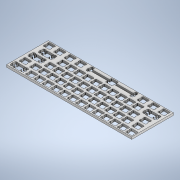
# Autodesk Inventor part: plate
Saved by Autodesk Inventor 2022 (Build 260153000, 153)
## iProperties
Created: 2022-03-01
Part Number: plate
Material: Generic
Document SubType Name: Modeling
Designer: Nathan Griffith
Density: 1 g/cm^3
Appearance: Default
Author: Nathan Griffith
Autodesk Inventor part; units mm, degrees
(part 1 of 2)
ref_plane "YZ Plane" through (0, 0, 0) normal (1, 0, 0) x (0, 1, 0)
ref_plane "XZ Plane" through (0, 0, 0) normal (0, 1, 0) x (-1, 0, 0)
ref_plane "XY Plane" through (0, 0, 0) normal (0, 0, 1) x (1, 0, 0)
sketch "Sketch1" plane through (0, 0, 0) normal (0, 1, 0) x (-1, 0, 0)
  line L0 (0.0951, 95.5075) -> (285.845, 95.5075)
  line L1 (285.845, 95.5075) -> (285.845, 0.2577)
  line L2 (285.845, 0.2577) -> (0.0951, 0.2577)
  line L3 (0.0951, 0.2577) -> (0.0951, 95.5075)
  line L4 (124.062, 16.7831) -> (124.062, 15.7827)
  line L5 (124.062, 15.7827) -> (123.263, 15.7827)
  line L6 (123.263, 15.7827) -> (123.263, 12.6848)
  line L7 (123.263, 12.6848) -> (124.062, 12.6848)
  line L8 (124.062, 12.6848) -> (124.062, 12.0826)
  line L9 (124.062, 12.0826) -> (84.4381, 12.0826)
  line L10 (84.4381, 12.0826) -> (84.4381, 15.3128)
  line L11 (84.4381, 15.3128) -> (82.7126, 15.3128)
  line L12 (82.7126, 15.3128) -> (82.7126, 16.2347)
  line L13 (82.7126, 16.2347) -> (79.412, 16.2347)
  line L14 (79.412, 16.2347) -> (79.412, 15.3128)
  line L15 (79.412, 15.3128) -> (77.687, 15.3128)
  line L16 (77.687, 15.3128) -> (77.687, 12.0826)
  line L17 (77.687, 12.0826) -> (76.8629, 12.0826)
  line L18 (76.8629, 12.0826) -> (76.8629, 9.2838)
  line L19 (76.8629, 9.2838) -> (77.687, 9.2838)
  line L20 (77.687, 9.2838) -> (77.687, 3.0138)
  line L21 (77.687, 3.0138) -> (79.412, 3.0138)
  line L22 (79.412, 3.0138) -> (79.412, 2.0326)
  line L23 (79.412, 2.0326) -> (82.7126, 2.0326)
  line L24 (82.7126, 2.0326) -> (82.7126, 3.0138)
  line L25 (82.7126, 3.0138) -> (84.4381, 3.0138)
  line L26 (84.4381, 3.0138) -> (84.4381, 7.4841)
  line L27 (84.4381, 7.4841) -> (124.062, 7.4841)
  line L28 (124.062, 7.4841) -> (124.062, 6.8833)
  line L29 (124.062, 6.8833) -> (123.263, 6.8833)
  line L30 (123.263, 6.8833) -> (123.263, 3.7827)
  line L31 (123.263, 3.7827) -> (124.062, 3.7827)
  line L32 (124.062, 3.7827) -> (124.062, 2.7836)
  line L33 (124.062, 2.7836) -> (138.063, 2.7836)
  line L34 (138.063, 2.7836) -> (138.063, 3.7827)
  line L35 (138.063, 3.7827) -> (138.862, 3.7827)
  line L36 (138.862, 3.7827) -> (138.862, 6.8833)
  line L37 (138.862, 6.8833) -> (138.063, 6.8833)
  line L38 (138.063, 6.8833) -> (138.063, 7.4841)
  line L39 (138.063, 7.4841) -> (177.687, 7.4841)
  line L40 (177.687, 7.4841) -> (177.687, 3.0138)
  line L41 (177.687, 3.0138) -> (179.412, 3.0138)
  line L42 (179.412, 3.0138) -> (179.412, 2.0326)
  line L43 (179.412, 2.0326) -> (182.713, 2.0326)
  line L44 (182.713, 2.0326) -> (182.713, 3.0138)
  line L45 (182.713, 3.0138) -> (184.438, 3.0138)
  line L46 (184.438, 3.0138) -> (184.438, 9.2838)
  line L47 (184.438, 9.2838) -> (185.262, 9.2838)
  line L48 (185.262, 9.2838) -> (185.262, 12.0826)
  line L49 (185.262, 12.0826) -> (184.438, 12.0826)
  line L50 (184.438, 12.0826) -> (184.438, 15.3128)
  line L51 (184.438, 15.3128) -> (182.713, 15.3128)
  line L52 (182.713, 15.3128) -> (182.713, 16.2347)
  line L53 (182.713, 16.2347) -> (179.412, 16.2347)
  line L54 (179.412, 16.2347) -> (179.412, 15.3128)
  line L55 (179.412, 15.3128) -> (177.687, 15.3128)
  line L56 (177.687, 15.3128) -> (177.687, 12.0826)
  line L57 (177.687, 12.0826) -> (138.063, 12.0826)
  line L58 (138.063, 12.0826) -> (138.063, 12.6848)
  line L59 (138.063, 12.6848) -> (138.862, 12.6848)
  line L60 (138.862, 12.6848) -> (138.862, 15.7827)
  line L61 (138.862, 15.7827) -> (138.063, 15.7827)
  line L62 (138.063, 15.7827) -> (138.063, 16.7831)
  line L63 (138.063, 16.7831) -> (124.062, 16.7831)
  line L64 (266.937, 16.7831) -> (266.937, 15.7827)
  line L65 (266.937, 15.7827) -> (266.138, 15.7827)
  line L66 (266.138, 15.7827) -> (266.138, 12.6848)
  line L67 (266.138, 12.6848) -> (266.937, 12.6848)
  line L68 (266.937, 12.6848) -> (266.937, 6.8833)
  line L69 (266.937, 6.8833) -> (266.138, 6.8833)
  line L70 (266.138, 6.8833) -> (266.138, 3.7827)
  line L71 (266.138, 3.7827) -> (266.937, 3.7827)
  line L72 (266.937, 3.7827) -> (266.937, 2.7836)
  line L73 (266.937, 2.7836) -> (280.938, 2.7836)
  line L74 (280.938, 2.7836) -> (280.938, 3.7827)
  line L75 (280.938, 3.7827) -> (281.737, 3.7827)
  line L76 (281.737, 3.7827) -> (281.737, 6.8833)
  line L77 (281.737, 6.8833) -> (280.938, 6.8833)
  line L78 (280.938, 6.8833) -> (280.938, 12.6848)
  line L79 (280.938, 12.6848) -> (281.737, 12.6848)
  line L80 (281.737, 12.6848) -> (281.737, 15.7827)
  line L81 (281.737, 15.7827) -> (280.938, 15.7827)
  line L82 (280.938, 15.7827) -> (280.938, 16.7831)
  line L83 (280.938, 16.7831) -> (266.937, 16.7831)
  line L84 (243.126, 16.7831) -> (243.126, 15.7827)
  line L85 (243.126, 15.7827) -> (242.325, 15.7827)
  line L86 (242.325, 15.7827) -> (242.325, 12.6848)
  line L87 (242.325, 12.6848) -> (243.126, 12.6848)
  line L88 (243.126, 12.6848) -> (243.126, 6.8833)
  line L89 (243.126, 6.8833) -> (242.325, 6.8833)
  line L90 (242.325, 6.8833) -> (242.325, 3.7827)
  line L91 (242.325, 3.7827) -> (243.126, 3.7827)
  line L92 (243.126, 3.7827) -> (243.126, 2.7836)
  line L93 (243.126, 2.7836) -> (257.125, 2.7836)
  line L94 (257.125, 2.7836) -> (257.125, 3.7827)
  line L95 (257.125, 3.7827) -> (257.926, 3.7827)
  line L96 (257.926, 3.7827) -> (257.926, 6.8833)
  line L97 (257.926, 6.8833) -> (257.125, 6.8833)
  line L98 (257.125, 6.8833) -> (257.125, 12.6848)
  line L99 (257.125, 12.6848) -> (257.926, 12.6848)
  line L100 (257.926, 12.6848) -> (257.926, 15.7827)
  line L101 (257.926, 15.7827) -> (257.125, 15.7827)
  line L102 (257.125, 15.7827) -> (257.125, 16.7831)
  line L103 (257.125, 16.7831) -> (243.126, 16.7831)
  line L104 (219.312, 16.7831) -> (219.312, 15.7827)
  line L105 (219.312, 15.7827) -> (218.513, 15.7827)
  line L106 (218.513, 15.7827) -> (218.513, 12.6848)
  line L107 (218.513, 12.6848) -> (219.312, 12.6848)
  line L108 (219.312, 12.6848) -> (219.312, 6.8833)
  line L109 (219.312, 6.8833) -> (218.513, 6.8833)
  line L110 (218.513, 6.8833) -> (218.513, 3.7827)
  line L111 (218.513, 3.7827) -> (219.312, 3.7827)
  line L112 (219.312, 3.7827) -> (219.312, 2.7836)
  line L113 (219.312, 2.7836) -> (233.313, 2.7836)
  line L114 (233.313, 2.7836) -> (233.313, 3.7827)
  line L115 (233.313, 3.7827) -> (234.112, 3.7827)
  line L116 (234.112, 3.7827) -> (234.112, 6.8833)
  line L117 (234.112, 6.8833) -> (233.313, 6.8833)
  line L118 (233.313, 6.8833) -> (233.313, 12.6848)
  line L119 (233.313, 12.6848) -> (234.112, 12.6848)
  line L120 (234.112, 12.6848) -> (234.112, 15.7827)
  line L121 (234.112, 15.7827) -> (233.313, 15.7827)
  line L122 (233.313, 15.7827) -> (233.313, 16.7831)
  line L123 (233.313, 16.7831) -> (219.312, 16.7831)
  line L124 (195.501, 16.7831) -> (195.501, 15.7827)
  line L125 (195.501, 15.7827) -> (194.7, 15.7827)
  line L126 (194.7, 15.7827) -> (194.7, 12.6848)
  line L127 (194.7, 12.6848) -> (195.501, 12.6848)
  line L128 (195.501, 12.6848) -> (195.501, 6.8833)
  line L129 (195.501, 6.8833) -> (194.7, 6.8833)
  line L130 (194.7, 6.8833) -> (194.7, 3.7827)
  line L131 (194.7, 3.7827) -> (195.501, 3.7827)
  line L132 (195.501, 3.7827) -> (195.501, 2.7836)
  line L133 (195.501, 2.7836) -> (209.5, 2.7836)
  line L134 (209.5, 2.7836) -> (209.5, 3.7827)
  line L135 (209.5, 3.7827) -> (210.301, 3.7827)
  line L136 (210.301, 3.7827) -> (210.301, 6.8833)
  line L137 (210.301, 6.8833) -> (209.5, 6.8833)
  line L138 (209.5, 6.8833) -> (209.5, 12.6848)
  line L139 (209.5, 12.6848) -> (210.301, 12.6848)
  line L140 (210.301, 12.6848) -> (210.301, 15.7827)
  line L141 (210.301, 15.7827) -> (209.5, 15.7827)
  line L142 (209.5, 15.7827) -> (209.5, 16.7831)
  line L143 (209.5, 16.7831) -> (195.501, 16.7831)
  line L144 (52.626, 16.7831) -> (52.626, 15.7827)
  line L145 (52.626, 15.7827) -> (51.8252, 15.7827)
  line L146 (51.8252, 15.7827) -> (51.8252, 12.6848)
  line L147 (51.8252, 12.6848) -> (52.626, 12.6848)
  line L148 (52.626, 12.6848) -> (52.626, 6.8833)
  line L149 (52.626, 6.8833) -> (51.8252, 6.8833)
  line L150 (51.8252, 6.8833) -> (51.8252, 3.7827)
  line L151 (51.8252, 3.7827) -> (52.626, 3.7827)
  line L152 (52.626, 3.7827) -> (52.626, 2.7836)
  line L153 (52.626, 2.7836) -> (66.6253, 2.7836)
  line L154 (66.6253, 2.7836) -> (66.6253, 3.7827)
  line L155 (66.6253, 3.7827) -> (67.4261, 3.7827)
  line L156 (67.4261, 3.7827) -> (67.4261, 6.8833)
  line L157 (67.4261, 6.8833) -> (66.6253, 6.8833)
  line L158 (66.6253, 6.8833) -> (66.6253, 12.6848)
  line L159 (66.6253, 12.6848) -> (67.4261, 12.6848)
  line L160 (67.4261, 12.6848) -> (67.4261, 15.7827)
  line L161 (67.4261, 15.7827) -> (66.6253, 15.7827)
  line L162 (66.6253, 15.7827) -> (66.6253, 16.7831)
  line L163 (66.6253, 16.7831) -> (52.626, 16.7831)
  line L164 (28.812, 16.7831) -> (28.812, 15.7827)
  line L165 (28.812, 15.7827) -> (28.0128, 15.7827)
  line L166 (28.0128, 15.7827) -> (28.0128, 12.6848)
  line L167 (28.0128, 12.6848) -> (28.812, 12.6848)
  line L168 (28.812, 12.6848) -> (28.812, 6.8833)
  line L169 (28.812, 6.8833) -> (28.0128, 6.8833)
  line L170 (28.0128, 6.8833) -> (28.0128, 3.7827)
  line L171 (28.0128, 3.7827) -> (28.812, 3.7827)
  line L172 (28.812, 3.7827) -> (28.812, 2.7836)
  line L173 (28.812, 2.7836) -> (42.8128, 2.7836)
  line L174 (42.8128, 2.7836) -> (42.8128, 3.7827)
  line L175 (42.8128, 3.7827) -> (43.6122, 3.7827)
  line L176 (43.6122, 3.7827) -> (43.6122, 6.8833)
  line L177 (43.6122, 6.8833) -> (42.8128, 6.8833)
  line L178 (42.8128, 6.8833) -> (42.8128, 12.6848)
  line L179 (42.8128, 12.6848) -> (43.6122, 12.6848)
  line L180 (43.6122, 12.6848) -> (43.6122, 15.7827)
  line L181 (43.6122, 15.7827) -> (42.8128, 15.7827)
  line L182 (42.8128, 15.7827) -> (42.8128, 16.7831)
  line L183 (42.8128, 16.7831) -> (28.812, 16.7831)
  line L184 (5.0009, 16.7831) -> (5.0009, 15.7827)
  line L185 (5.0009, 15.7827) -> (4.2003, 15.7827)
  line L186 (4.2003, 15.7827) -> (4.2003, 12.6848)
  line L187 (4.2003, 12.6848) -> (5.0009, 12.6848)
  line L188 (5.0009, 12.6848) -> (5.0009, 6.8833)
  line L189 (5.0009, 6.8833) -> (4.2003, 6.8833)
  line L190 (4.2003, 6.8833) -> (4.2003, 3.7827)
  line L191 (4.2003, 3.7827) -> (5.0009, 3.7827)
  line L192 (5.0009, 3.7827) -> (5.0009, 2.7836)
  line L193 (5.0009, 2.7836) -> (19.0004, 2.7836)
  line L194 (19.0004, 2.7836) -> (19.0004, 3.7827)
  line L195 (19.0004, 3.7827) -> (19.801, 3.7827)
  line L196 (19.801, 3.7827) -> (19.801, 6.8833)
  line L197 (19.801, 6.8833) -> (19.0004, 6.8833)
  line L198 (19.0004, 6.8833) -> (19.0004, 12.6848)
  line L199 (19.0004, 12.6848) -> (19.801, 12.6848)
  line L200 (19.801, 12.6848) -> (19.801, 15.7827)
  line L201 (19.801, 15.7827) -> (19.0004, 15.7827)
  line L202 (19.0004, 15.7827) -> (19.0004, 16.7831)
  line L203 (19.0004, 16.7831) -> (5.0009, 16.7831)
  line L204 (252.65, 35.833) -> (252.65, 34.8327)
  line L205 (252.65, 34.8327) -> (251.849, 34.8327)
  line L206 (251.849, 34.8327) -> (251.849, 31.7348)
  line L207 (251.849, 31.7348) -> (252.65, 31.7348)
  line L208 (252.65, 31.7348) -> (252.65, 31.1326)
  line L209 (252.65, 31.1326) -> (251.126, 31.1326)
  line L210 (251.126, 31.1326) -> (251.126, 34.3628)
  line L211 (251.126, 34.3628) -> (249.4, 34.3628)
  line L212 (249.4, 34.3628) -> (249.4, 35.2848)
  line L213 (249.4, 35.2848) -> (246.101, 35.2848)
  line L214 (246.101, 35.2848) -> (246.101, 34.3628)
  line L215 (246.101, 34.3628) -> (244.376, 34.3628)
  line L216 (244.376, 34.3628) -> (244.376, 31.1326)
  line L217 (244.376, 31.1326) -> (243.55, 31.1326)
  line L218 (243.55, 31.1326) -> (243.55, 28.3338)
  line L219 (243.55, 28.3338) -> (244.376, 28.3338)
  line L220 (244.376, 28.3338) -> (244.376, 22.0638)
  line L221 (244.376, 22.0638) -> (246.101, 22.0638)
  line L222 (246.101, 22.0638) -> (246.101, 21.0826)
  line L223 (246.101, 21.0826) -> (249.4, 21.0826)
  line L224 (249.4, 21.0826) -> (249.4, 22.0638)
  line L225 (249.4, 22.0638) -> (251.126, 22.0638)
  line L226 (251.126, 22.0638) -> (251.126, 26.5327)
  line L227 (251.126, 26.5327) -> (252.65, 26.5327)
  line L228 (252.65, 26.5327) -> (252.65, 25.9333)
  line L229 (252.65, 25.9333) -> (251.849, 25.9333)
  line L230 (251.849, 25.9333) -> (251.849, 22.8327)
  line L231 (251.849, 22.8327) -> (252.65, 22.8327)
  line L232 (252.65, 22.8327) -> (252.65, 21.8336)
  line L233 (252.65, 21.8336) -> (266.65, 21.8336)
  line L234 (266.65, 21.8336) -> (266.65, 22.8327)
  line L235 (266.65, 22.8327) -> (267.451, 22.8327)
  line L236 (267.451, 22.8327) -> (267.451, 25.9333)
  line L237 (267.451, 25.9333) -> (266.65, 25.9333)
  line L238 (266.65, 25.9333) -> (266.65, 26.5327)
  line L239 (266.65, 26.5327) -> (268.176, 26.5327)
  line L240 (268.176, 26.5327) -> (268.176, 22.0638)
  line L241 (268.176, 22.0638) -> (269.9, 22.0638)
  line L242 (269.9, 22.0638) -> (269.9, 21.0826)
  line L243 (269.9, 21.0826) -> (273.2, 21.0826)
  line L244 (273.2, 21.0826) -> (273.2, 22.0638)
  line L245 (273.2, 22.0638) -> (274.925, 22.0638)
  line L246 (274.925, 22.0638) -> (274.925, 28.3338)
  line L247 (274.925, 28.3338) -> (275.751, 28.3338)
  line L248 (275.751, 28.3338) -> (275.751, 31.1326)
  line L249 (275.751, 31.1326) -> (274.925, 31.1326)
  line L250 (274.925, 31.1326) -> (274.925, 34.3628)
  line L251 (274.925, 34.3628) -> (273.2, 34.3628)
  line L252 (273.2, 34.3628) -> (273.2, 35.2848)
  line L253 (273.2, 35.2848) -> (269.9, 35.2848)
  line L254 (269.9, 35.2848) -> (269.9, 34.3628)
  line L255 (269.9, 34.3628) -> (268.176, 34.3628)
  line L256 (268.176, 34.3628) -> (268.176, 31.1326)
  line L257 (268.176, 31.1326) -> (266.65, 31.1326)
  line L258 (266.65, 31.1326) -> (266.65, 31.7348)
  line L259 (266.65, 31.7348) -> (267.451, 31.7348)
  line L260 (267.451, 31.7348) -> (267.451, 34.8327)
  line L261 (267.451, 34.8327) -> (266.65, 34.8327)
  line L262 (266.65, 34.8327) -> (266.65, 35.833)
  line L263 (266.65, 35.833) -> (252.65, 35.833)
  line L264 (14.5259, 35.833) -> (14.5259, 34.8327)
  line L265 (14.5259, 34.8327) -> (13.7253, 34.8327)
  line L266 (13.7253, 34.8327) -> (13.7253, 31.7348)
  line L267 (13.7253, 31.7348) -> (14.5259, 31.7348)
  line L268 (14.5259, 31.7348) -> (14.5259, 31.1326)
  line L269 (14.5259, 31.1326) -> (13.0004, 31.1326)
  line L270 (13.0004, 31.1326) -> (13.0004, 34.3628)
  line L271 (13.0004, 34.3628) -> (11.2751, 34.3628)
  line L272 (11.2751, 34.3628) -> (11.2751, 35.2848)
  line L273 (11.2751, 35.2848) -> (7.9761, 35.2848)
  line L274 (7.9761, 35.2848) -> (7.9761, 34.3628)
  line L275 (7.9761, 34.3628) -> (6.2508, 34.3628)
  line L276 (6.2508, 34.3628) -> (6.2508, 31.1326)
  line L277 (6.2508, 31.1326) -> (5.4253, 31.1326)
  line L278 (5.4253, 31.1326) -> (5.4253, 28.3338)
  line L279 (5.4253, 28.3338) -> (6.2508, 28.3338)
  line L280 (6.2508, 28.3338) -> (6.2508, 22.0638)
  line L281 (6.2508, 22.0638) -> (7.9761, 22.0638)
  line L282 (7.9761, 22.0638) -> (7.9761, 21.0826)
  line L283 (7.9761, 21.0826) -> (11.2751, 21.0826)
  line L284 (11.2751, 21.0826) -> (11.2751, 22.0638)
  line L285 (11.2751, 22.0638) -> (13.0004, 22.0638)
  line L286 (13.0004, 22.0638) -> (13.0004, 26.5327)
  line L287 (13.0004, 26.5327) -> (14.5259, 26.5327)
  line L288 (14.5259, 26.5327) -> (14.5259, 25.9333)
  line L289 (14.5259, 25.9333) -> (13.7253, 25.9333)
  line L290 (13.7253, 25.9333) -> (13.7253, 22.8327)
  line L291 (13.7253, 22.8327) -> (14.5259, 22.8327)
  line L292 (14.5259, 22.8327) -> (14.5259, 21.8336)
  line L293 (14.5259, 21.8336) -> (28.5254, 21.8336)
  line L294 (28.5254, 21.8336) -> (28.5254, 22.8327)
  line L295 (28.5254, 22.8327) -> (29.326, 22.8327)
  line L296 (29.326, 22.8327) -> (29.326, 25.9333)
  line L297 (29.326, 25.9333) -> (28.5254, 25.9333)
  line L298 (28.5254, 25.9333) -> (28.5254, 26.5327)
  line L299 (28.5254, 26.5327) -> (30.0509, 26.5327)
  line L300 (30.0509, 26.5327) -> (30.0509, 22.0638)
  line L301 (30.0509, 22.0638) -> (31.7748, 22.0638)
  line L302 (31.7748, 22.0638) -> (31.7748, 21.0826)
  line L303 (31.7748, 21.0826) -> (35.0752, 21.0826)
  line L304 (35.0752, 21.0826) -> (35.0752, 22.0638)
  line L305 (35.0752, 22.0638) -> (36.8004, 22.0638)
  line L306 (36.8004, 22.0638) -> (36.8004, 28.3338)
  line L307 (36.8004, 28.3338) -> (37.6259, 28.3338)
  line L308 (37.6259, 28.3338) -> (37.6259, 31.1326)
  line L309 (37.6259, 31.1326) -> (36.8004, 31.1326)
  line L310 (36.8004, 31.1326) -> (36.8004, 34.3628)
  line L311 (36.8004, 34.3628) -> (35.0752, 34.3628)
  line L312 (35.0752, 34.3628) -> (35.0752, 35.2848)
  line L313 (35.0752, 35.2848) -> (31.7748, 35.2848)
  line L314 (31.7748, 35.2848) -> (31.7748, 34.3628)
  line L315 (31.7748, 34.3628) -> (30.0509, 34.3628)
  line L316 (30.0509, 34.3628) -> (30.0509, 31.1326)
  line L317 (30.0509, 31.1326) -> (28.5254, 31.1326)
  line L318 (28.5254, 31.1326) -> (28.5254, 31.7348)
  line L319 (28.5254, 31.7348) -> (29.326, 31.7348)
  line L320 (29.326, 31.7348) -> (29.326, 34.8327)
  line L321 (29.326, 34.8327) -> (28.5254, 34.8327)
  line L322 (28.5254, 34.8327) -> (28.5254, 35.833)
  line L323 (28.5254, 35.833) -> (14.5259, 35.833)
  line L324 (216.932, 35.833) -> (216.932, 34.8327)
  line L325 (216.932, 34.8327) -> (216.131, 34.8327)
  line L326 (216.131, 34.8327) -> (216.131, 31.7348)
  line L327 (216.131, 31.7348) -> (216.932, 31.7348)
  line L328 (216.932, 31.7348) -> (216.932, 25.9333)
  line L329 (216.932, 25.9333) -> (216.131, 25.9333)
  line L330 (216.131, 25.9333) -> (216.131, 22.8327)
  line L331 (216.131, 22.8327) -> (216.932, 22.8327)
  line L332 (216.932, 22.8327) -> (216.932, 21.8336)
  line L333 (216.932, 21.8336) -> (230.932, 21.8336)
  line L334 (230.932, 21.8336) -> (230.932, 22.8327)
  line L335 (230.932, 22.8327) -> (231.731, 22.8327)
  line L336 (231.731, 22.8327) -> (231.731, 25.9333)
  line L337 (231.731, 25.9333) -> (230.932, 25.9333)
  line L338 (230.932, 25.9333) -> (230.932, 31.7348)
  line L339 (230.932, 31.7348) -> (231.731, 31.7348)
  line L340 (231.731, 31.7348) -> (231.731, 34.8327)
  line L341 (231.731, 34.8327) -> (230.932, 34.8327)
  line L342 (230.932, 34.8327) -> (230.932, 35.833)
  line L343 (230.932, 35.833) -> (216.932, 35.833)
  line L344 (197.882, 35.833) -> (197.882, 34.8327)
  line L345 (197.882, 34.8327) -> (197.081, 34.8327)
  line L346 (197.081, 34.8327) -> (197.081, 31.7348)
  line L347 (197.081, 31.7348) -> (197.882, 31.7348)
  line L348 (197.882, 31.7348) -> (197.882, 25.9333)
  line L349 (197.882, 25.9333) -> (197.081, 25.9333)
  line L350 (197.081, 25.9333) -> (197.081, 22.8327)
  line L351 (197.081, 22.8327) -> (197.882, 22.8327)
  line L352 (197.882, 22.8327) -> (197.882, 21.8336)
  line L353 (197.882, 21.8336) -> (211.882, 21.8336)
  line L354 (211.882, 21.8336) -> (211.882, 22.8327)
  line L355 (211.882, 22.8327) -> (212.681, 22.8327)
  line L356 (212.681, 22.8327) -> (212.681, 25.9333)
  line L357 (212.681, 25.9333) -> (211.882, 25.9333)
  line L358 (211.882, 25.9333) -> (211.882, 31.7348)
  line L359 (211.882, 31.7348) -> (212.681, 31.7348)
  line L360 (212.681, 31.7348) -> (212.681, 34.8327)
  line L361 (212.681, 34.8327) -> (211.882, 34.8327)
  line L362 (211.882, 34.8327) -> (211.882, 35.833)
  line L363 (211.882, 35.833) -> (197.882, 35.833)
  line L364 (178.832, 35.833) -> (178.832, 34.8327)
  line L365 (178.832, 34.8327) -> (178.031, 34.8327)
  line L366 (178.031, 34.8327) -> (178.031, 31.7348)
  line L367 (178.031, 31.7348) -> (178.832, 31.7348)
  line L368 (178.832, 31.7348) -> (178.832, 25.9333)
  line L369 (178.832, 25.9333) -> (178.031, 25.9333)
  line L370 (178.031, 25.9333) -> (178.031, 22.8327)
  line L371 (178.031, 22.8327) -> (178.832, 22.8327)
  line L372 (178.832, 22.8327) -> (178.832, 21.8336)
  line L373 (178.832, 21.8336) -> (192.832, 21.8336)
  line L374 (192.832, 21.8336) -> (192.832, 22.8327)
  line L375 (192.832, 22.8327) -> (193.631, 22.8327)
  line L376 (193.631, 22.8327) -> (193.631, 25.9333)
  line L377 (193.631, 25.9333) -> (192.832, 25.9333)
  line L378 (192.832, 25.9333) -> (192.832, 31.7348)
  line L379 (192.832, 31.7348) -> (193.631, 31.7348)
  line L380 (193.631, 31.7348) -> (193.631, 34.8327)
  line L381 (193.631, 34.8327) -> (192.832, 34.8327)
  line L382 (192.832, 34.8327) -> (192.832, 35.833)
  line L383 (192.832, 35.833) -> (178.832, 35.833)
  line L384 (159.782, 35.833) -> (159.782, 34.8327)
  line L385 (159.782, 34.8327) -> (158.981, 34.8327)
  line L386 (158.981, 34.8327) -> (158.981, 31.7348)
  line L387 (158.981, 31.7348) -> (159.782, 31.7348)
  line L388 (159.782, 31.7348) -> (159.782, 25.9333)
  line L389 (159.782, 25.9333) -> (158.981, 25.9333)
  line L390 (158.981, 25.9333) -> (158.981, 22.8327)
  line L391 (158.981, 22.8327) -> (159.782, 22.8327)
  line L392 (159.782, 22.8327) -> (159.782, 21.8336)
  line L393 (159.782, 21.8336) -> (173.782, 21.8336)
  line L394 (173.782, 21.8336) -> (173.782, 22.8327)
  line L395 (173.782, 22.8327) -> (174.581, 22.8327)
  line L396 (174.581, 22.8327) -> (174.581, 25.9333)
  line L397 (174.581, 25.9333) -> (173.782, 25.9333)
  line L398 (173.782, 25.9333) -> (173.782, 31.7348)
  line L399 (173.782, 31.7348) -> (174.581, 31.7348)
  line L400 (174.581, 31.7348) -> (174.581, 34.8327)
  line L401 (174.581, 34.8327) -> (173.782, 34.8327)
  line L402 (173.782, 34.8327) -> (173.782, 35.833)
  line L403 (173.782, 35.833) -> (159.782, 35.833)
  line L404 (140.732, 35.833) -> (140.732, 34.8327)
  line L405 (140.732, 34.8327) -> (139.931, 34.8327)
  line L406 (139.931, 34.8327) -> (139.931, 31.7348)
  line L407 (139.931, 31.7348) -> (140.732, 31.7348)
  line L408 (140.732, 31.7348) -> (140.732, 25.9333)
  line L409 (140.732, 25.9333) -> (139.931, 25.9333)
  line L410 (139.931, 25.9333) -> (139.931, 22.8327)
  line L411 (139.931, 22.8327) -> (140.732, 22.8327)
  line L412 (140.732, 22.8327) -> (140.732, 21.8336)
  line L413 (140.732, 21.8336) -> (154.732, 21.8336)
  line L414 (154.732, 21.8336) -> (154.732, 22.8327)
  line L415 (154.732, 22.8327) -> (155.531, 22.8327)
  line L416 (155.531, 22.8327) -> (155.531, 25.9333)
  line L417 (155.531, 25.9333) -> (154.732, 25.9333)
  line L418 (154.732, 25.9333) -> (154.732, 31.7348)
  line L419 (154.732, 31.7348) -> (155.531, 31.7348)
  line L420 (155.531, 31.7348) -> (155.531, 34.8327)
  line L421 (155.531, 34.8327) -> (154.732, 34.8327)
  line L422 (154.732, 34.8327) -> (154.732, 35.833)
  line L423 (154.732, 35.833) -> (140.732, 35.833)
  line L424 (121.682, 35.833) -> (121.682, 34.8327)
  line L425 (121.682, 34.8327) -> (120.881, 34.8327)
  line L426 (120.881, 34.8327) -> (120.881, 31.7348)
  line L427 (120.881, 31.7348) -> (121.682, 31.7348)
  line L428 (121.682, 31.7348) -> (121.682, 25.9333)
  line L429 (121.682, 25.9333) -> (120.881, 25.9333)
  line L430 (120.881, 25.9333) -> (120.881, 22.8327)
  line L431 (120.881, 22.8327) -> (121.682, 22.8327)
  line L432 (121.682, 22.8327) -> (121.682, 21.8336)
  line L433 (121.682, 21.8336) -> (135.682, 21.8336)
  line L434 (135.682, 21.8336) -> (135.682, 22.8327)
  line L435 (135.682, 22.8327) -> (136.481, 22.8327)
  line L436 (136.481, 22.8327) -> (136.481, 25.9333)
  line L437 (136.481, 25.9333) -> (135.682, 25.9333)
  line L438 (135.682, 25.9333) -> (135.682, 31.7348)
  line L439 (135.682, 31.7348) -> (136.481, 31.7348)
  line L440 (136.481, 31.7348) -> (136.481, 34.8327)
  line L441 (136.481, 34.8327) -> (135.682, 34.8327)
  line L442 (135.682, 34.8327) -> (135.682, 35.833)
  line L443 (135.682, 35.833) -> (121.682, 35.833)
  line L444 (102.632, 35.833) -> (102.632, 34.8327)
  line L445 (102.632, 34.8327) -> (101.831, 34.8327)
  line L446 (101.831, 34.8327) -> (101.831, 31.7348)
  line L447 (101.831, 31.7348) -> (102.632, 31.7348)
  line L448 (102.632, 31.7348) -> (102.632, 25.9333)
  line L449 (102.632, 25.9333) -> (101.831, 25.9333)
  line L450 (101.831, 25.9333) -> (101.831, 22.8327)
  line L451 (101.831, 22.8327) -> (102.632, 22.8327)
  line L452 (102.632, 22.8327) -> (102.632, 21.8336)
  line L453 (102.632, 21.8336) -> (116.632, 21.8336)
  line L454 (116.632, 21.8336) -> (116.632, 22.8327)
  line L455 (116.632, 22.8327) -> (117.431, 22.8327)
  line L456 (117.431, 22.8327) -> (117.431, 25.9333)
  line L457 (117.431, 25.9333) -> (116.632, 25.9333)
  line L458 (116.632, 25.9333) -> (116.632, 31.7348)
  line L459 (116.632, 31.7348) -> (117.431, 31.7348)
  line L460 (117.431, 31.7348) -> (117.431, 34.8327)
  line L461 (117.431, 34.8327) -> (116.632, 34.8327)
  line L462 (116.632, 34.8327) -> (116.632, 35.833)
  line L463 (116.632, 35.833) -> (102.632, 35.833)
  line L464 (83.5822, 35.833) -> (83.5822, 34.8327)
  line L465 (83.5822, 34.8327) -> (82.7814, 34.8327)
  line L466 (82.7814, 34.8327) -> (82.7814, 31.7348)
  line L467 (82.7814, 31.7348) -> (83.5822, 31.7348)
  line L468 (83.5822, 31.7348) -> (83.5822, 25.9333)
  line L469 (83.5822, 25.9333) -> (82.7814, 25.9333)
  line L470 (82.7814, 25.9333) -> (82.7814, 22.8327)
  line L471 (82.7814, 22.8327) -> (83.5822, 22.8327)
  line L472 (83.5822, 22.8327) -> (83.5822, 21.8336)
  line L473 (83.5822, 21.8336) -> (97.5815, 21.8336)
  line L474 (97.5815, 21.8336) -> (97.5815, 22.8327)
  line L475 (97.5815, 22.8327) -> (98.3809, 22.8327)
  line L476 (98.3809, 22.8327) -> (98.3809, 25.9333)
  line L477 (98.3809, 25.9333) -> (97.5815, 25.9333)
  line L478 (97.5815, 25.9333) -> (97.5815, 31.7348)
  line L479 (97.5815, 31.7348) -> (98.3809, 31.7348)
  line L480 (98.3809, 31.7348) -> (98.3809, 34.8327)
  line L481 (98.3809, 34.8327) -> (97.5815, 34.8327)
  line L482 (97.5815, 34.8327) -> (97.5815, 35.833)
  line L483 (97.5815, 35.833) -> (83.5822, 35.833)
  line L484 (64.5322, 35.833) -> (64.5322, 34.8327)
  line L485 (64.5322, 34.8327) -> (63.7314, 34.8327)
  line L486 (63.7314, 34.8327) -> (63.7314, 31.7348)
  line L487 (63.7314, 31.7348) -> (64.5322, 31.7348)
  line L488 (64.5322, 31.7348) -> (64.5322, 25.9333)
  line L489 (64.5322, 25.9333) -> (63.7314, 25.9333)
  line L490 (63.7314, 25.9333) -> (63.7314, 22.8327)
  line L491 (63.7314, 22.8327) -> (64.5322, 22.8327)
  line L492 (64.5322, 22.8327) -> (64.5322, 21.8336)
  line L493 (64.5322, 21.8336) -> (78.5315, 21.8336)
  line L494 (78.5315, 21.8336) -> (78.5315, 22.8327)
  line L495 (78.5315, 22.8327) -> (79.3309, 22.8327)
  line L496 (79.3309, 22.8327) -> (79.3309, 25.9333)
  line L497 (79.3309, 25.9333) -> (78.5315, 25.9333)
  line L498 (78.5315, 25.9333) -> (78.5315, 31.7348)
  line L499 (78.5315, 31.7348) -> (79.3309, 31.7348)
  line L500 (79.3309, 31.7348) -> (79.3309, 34.8327)
  line L501 (79.3309, 34.8327) -> (78.5315, 34.8327)
  line L502 (78.5315, 34.8327) -> (78.5315, 35.833)
  line L503 (78.5315, 35.833) -> (64.5322, 35.833)
  line L504 (45.4822, 35.833) -> (45.4822, 34.8327)
  line L505 (45.4822, 34.8327) -> (44.6814, 34.8327)
  line L506 (44.6814, 34.8327) -> (44.6814, 31.7348)
  line L507 (44.6814, 31.7348) -> (45.4822, 31.7348)
  line L508 (45.4822, 31.7348) -> (45.4822, 25.9333)
  line L509 (45.4822, 25.9333) -> (44.6814, 25.9333)
  line L510 (44.6814, 25.9333) -> (44.6814, 22.8327)
  line L511 (44.6814, 22.8327) -> (45.4822, 22.8327)
  line L512 (45.4822, 22.8327) -> (45.4822, 21.8336)
  line L513 (45.4822, 21.8336) -> (59.4815, 21.8336)
  line L514 (59.4815, 21.8336) -> (59.4815, 22.8327)
  line L515 (59.4815, 22.8327) -> (60.2809, 22.8327)
  line L516 (60.2809, 22.8327) -> (60.2809, 25.9333)
  line L517 (60.2809, 25.9333) -> (59.4815, 25.9333)
  line L518 (59.4815, 25.9333) -> (59.4815, 31.7348)
  line L519 (59.4815, 31.7348) -> (60.2809, 31.7348)
  line L520 (60.2809, 31.7348) -> (60.2809, 34.8327)
  line L521 (60.2809, 34.8327) -> (59.4815, 34.8327)
  line L522 (59.4815, 34.8327) -> (59.4815, 35.833)
  line L523 (59.4815, 35.833) -> (45.4822, 35.833)
  line L524 (257.412, 54.8831) -> (257.412, 53.8826)
  line L525 (257.412, 53.8826) -> (256.611, 53.8826)
  line L526 (256.611, 53.8826) -> (256.611, 50.7834)
  line L527 (256.611, 50.7834) -> (257.412, 50.7834)
  line L528 (257.412, 50.7834) -> (257.412, 50.1826)
  line L529 (257.412, 50.1826) -> (255.888, 50.1826)
  line L530 (255.888, 50.1826) -> (255.888, 53.4127)
  line L531 (255.888, 53.4127) -> (254.161, 53.4127)
  line L532 (254.161, 53.4127) -> (254.161, 54.3334)
  line L533 (254.161, 54.3334) -> (250.862, 54.3334)
  line L534 (250.862, 54.3334) -> (250.862, 53.4127)
  line L535 (250.862, 53.4127) -> (249.137, 53.4127)
  line L536 (249.137, 53.4127) -> (249.137, 50.1826)
  line L537 (249.137, 50.1826) -> (248.313, 50.1826)
  line L538 (248.313, 50.1826) -> (248.313, 47.3837)
  line L539 (248.313, 47.3837) -> (249.137, 47.3837)
  line L540 (249.137, 47.3837) -> (249.137, 41.1138)
  line L541 (249.137, 41.1138) -> (250.862, 41.1138)
  line L542 (250.862, 41.1138) -> (250.862, 40.1327)
  line L543 (250.862, 40.1327) -> (254.161, 40.1327)
  line L544 (254.161, 40.1327) -> (254.161, 41.1138)
  line L545 (254.161, 41.1138) -> (255.888, 41.1138)
  line L546 (255.888, 41.1138) -> (255.888, 45.5828)
  line L547 (255.888, 45.5828) -> (257.412, 45.5828)
  line L548 (257.412, 45.5828) -> (257.412, 44.9834)
  line L549 (257.412, 44.9834) -> (256.611, 44.9834)
  line L550 (256.611, 44.9834) -> (256.611, 41.8828)
  line L551 (256.611, 41.8828) -> (257.412, 41.8828)
  line L552 (257.412, 41.8828) -> (257.412, 40.8838)
  line L553 (257.412, 40.8838) -> (271.413, 40.8838)
  line L554 (271.413, 40.8838) -> (271.413, 41.8828)
  line L555 (271.413, 41.8828) -> (272.212, 41.8828)
  line L556 (272.212, 41.8828) -> (272.212, 44.9834)
  line L557 (272.212, 44.9834) -> (271.413, 44.9834)
  line L558 (271.413, 44.9834) -> (271.413, 45.5828)
  line L559 (271.413, 45.5828) -> (272.937, 45.5828)
  line L560 (272.937, 45.5828) -> (272.937, 41.1138)
  line L561 (272.937, 41.1138) -> (274.662, 41.1138)
  line L562 (274.662, 41.1138) -> (274.662, 40.1327)
  line L563 (274.662, 40.1327) -> (277.963, 40.1327)
  line L564 (277.963, 40.1327) -> (277.963, 41.1138)
  line L565 (277.963, 41.1138) -> (279.688, 41.1138)
  line L566 (279.688, 41.1138) -> (279.688, 47.3837)
  line L567 (279.688, 47.3837) -> (280.512, 47.3837)
  line L568 (280.512, 47.3837) -> (280.512, 50.1826)
  line L569 (280.512, 50.1826) -> (279.688, 50.1826)
  line L570 (279.688, 50.1826) -> (279.688, 53.4127)
  line L571 (279.688, 53.4127) -> (277.963, 53.4127)
  line L572 (277.963, 53.4127) -> (277.963, 54.3334)
  line L573 (277.963, 54.3334) -> (274.662, 54.3334)
  line L574 (274.662, 54.3334) -> (274.662, 53.4127)
  line L575 (274.662, 53.4127) -> (272.937, 53.4127)
  line L576 (272.937, 53.4127) -> (272.937, 50.1826)
  line L577 (272.937, 50.1826) -> (271.413, 50.1826)
  line L578 (271.413, 50.1826) -> (271.413, 50.7834)
  line L579 (271.413, 50.7834) -> (272.212, 50.7834)
  line L580 (272.212, 50.7834) -> (272.212, 53.8826)
  line L581 (272.212, 53.8826) -> (271.413, 53.8826)
  line L582 (271.413, 53.8826) -> (271.413, 54.8831)
  line L583 (271.413, 54.8831) -> (257.412, 54.8831)
  line L584 (226.457, 54.8831) -> (226.457, 53.8826)
  line L585 (226.457, 53.8826) -> (225.656, 53.8826)
  line L586 (225.656, 53.8826) -> (225.656, 50.7834)
  line L587 (225.656, 50.7834) -> (226.457, 50.7834)
  line L588 (226.457, 50.7834) -> (226.457, 44.9834)
  line L589 (226.457, 44.9834) -> (225.656, 44.9834)
  line L590 (225.656, 44.9834) -> (225.656, 41.8828)
  line L591 (225.656, 41.8828) -> (226.457, 41.8828)
  line L592 (226.457, 41.8828) -> (226.457, 40.8838)
  line L593 (226.457, 40.8838) -> (240.457, 40.8838)
  line L594 (240.457, 40.8838) -> (240.457, 41.8828)
  line L595 (240.457, 41.8828) -> (241.256, 41.8828)
  line L596 (241.256, 41.8828) -> (241.256, 44.9834)
  line L597 (241.256, 44.9834) -> (240.457, 44.9834)
  line L598 (240.457, 44.9834) -> (240.457, 50.7834)
  line L599 (240.457, 50.7834) -> (241.256, 50.7834)
  line L600 (241.256, 50.7834) -> (241.256, 53.8826)
  line L601 (241.256, 53.8826) -> (240.457, 53.8826)
  line L602 (240.457, 53.8826) -> (240.457, 54.8831)
  line L603 (240.457, 54.8831) -> (226.457, 54.8831)
  line L604 (207.407, 54.8831) -> (207.407, 53.8826)
  line L605 (207.407, 53.8826) -> (206.606, 53.8826)
  line L606 (206.606, 53.8826) -> (206.606, 50.7834)
  line L607 (206.606, 50.7834) -> (207.407, 50.7834)
  line L608 (207.407, 50.7834) -> (207.407, 44.9834)
  line L609 (207.407, 44.9834) -> (206.606, 44.9834)
  line L610 (206.606, 44.9834) -> (206.606, 41.8828)
  line L611 (206.606, 41.8828) -> (207.407, 41.8828)
  line L612 (207.407, 41.8828) -> (207.407, 40.8838)
  line L613 (207.407, 40.8838) -> (221.407, 40.8838)
  line L614 (221.407, 40.8838) -> (221.407, 41.8828)
  line L615 (221.407, 41.8828) -> (222.206, 41.8828)
  line L616 (222.206, 41.8828) -> (222.206, 44.9834)
  line L617 (222.206, 44.9834) -> (221.407, 44.9834)
  line L618 (221.407, 44.9834) -> (221.407, 50.7834)
  line L619 (221.407, 50.7834) -> (222.206, 50.7834)
  line L620 (222.206, 50.7834) -> (222.206, 53.8826)
  line L621 (222.206, 53.8826) -> (221.407, 53.8826)
  line L622 (221.407, 53.8826) -> (221.407, 54.8831)
  line L623 (221.407, 54.8831) -> (207.407, 54.8831)
  line L624 (188.357, 54.8831) -> (188.357, 53.8826)
  line L625 (188.357, 53.8826) -> (187.556, 53.8826)
  line L626 (187.556, 53.8826) -> (187.556, 50.7834)
  line L627 (187.556, 50.7834) -> (188.357, 50.7834)
  line L628 (188.357, 50.7834) -> (188.357, 44.9834)
  line L629 (188.357, 44.9834) -> (187.556, 44.9834)
  line L630 (187.556, 44.9834) -> (187.556, 41.8828)
  line L631 (187.556, 41.8828) -> (188.357, 41.8828)
  line L632 (188.357, 41.8828) -> (188.357, 40.8838)
  line L633 (188.357, 40.8838) -> (202.357, 40.8838)
  line L634 (202.357, 40.8838) -> (202.357, 41.8828)
  line L635 (202.357, 41.8828) -> (203.156, 41.8828)
  line L636 (203.156, 41.8828) -> (203.156, 44.9834)
  line L637 (203.156, 44.9834) -> (202.357, 44.9834)
  line L638 (202.357, 44.9834) -> (202.357, 50.7834)
  line L639 (202.357, 50.7834) -> (203.156, 50.7834)
  line L640 (203.156, 50.7834) -> (203.156, 53.8826)
  line L641 (203.156, 53.8826) -> (202.357, 53.8826)
  line L642 (202.357, 53.8826) -> (202.357, 54.8831)
  line L643 (202.357, 54.8831) -> (188.357, 54.8831)
  line L644 (169.307, 54.8831) -> (169.307, 53.8826)
  line L645 (169.307, 53.8826) -> (168.506, 53.8826)
  line L646 (168.506, 53.8826) -> (168.506, 50.7834)
  line L647 (168.506, 50.7834) -> (169.307, 50.7834)
  line L648 (169.307, 50.7834) -> (169.307, 44.9834)
  line L649 (169.307, 44.9834) -> (168.506, 44.9834)
  line L650 (168.506, 44.9834) -> (168.506, 41.8828)
  line L651 (168.506, 41.8828) -> (169.307, 41.8828)
  line L652 (169.307, 41.8828) -> (169.307, 40.8838)
  line L653 (169.307, 40.8838) -> (183.307, 40.8838)
  line L654 (183.307, 40.8838) -> (183.307, 41.8828)
  line L655 (183.307, 41.8828) -> (184.106, 41.8828)
  line L656 (184.106, 41.8828) -> (184.106, 44.9834)
  line L657 (184.106, 44.9834) -> (183.307, 44.9834)
  line L658 (183.307, 44.9834) -> (183.307, 50.7834)
  line L659 (183.307, 50.7834) -> (184.106, 50.7834)
  line L660 (184.106, 50.7834) -> (184.106, 53.8826)
  line L661 (184.106, 53.8826) -> (183.307, 53.8826)
  line L662 (183.307, 53.8826) -> (183.307, 54.8831)
  line L663 (183.307, 54.8831) -> (169.307, 54.8831)
  line L664 (150.257, 54.8831) -> (150.257, 53.8826)
  line L665 (150.257, 53.8826) -> (149.456, 53.8826)
  line L666 (149.456, 53.8826) -> (149.456, 50.7834)
  line L667 (149.456, 50.7834) -> (150.257, 50.7834)
  line L668 (150.257, 50.7834) -> (150.257, 44.9834)
  line L669 (150.257, 44.9834) -> (149.456, 44.9834)
  line L670 (149.456, 44.9834) -> (149.456, 41.8828)
  line L671 (149.456, 41.8828) -> (150.257, 41.8828)
  line L672 (150.257, 41.8828) -> (150.257, 40.8838)
  line L673 (150.257, 40.8838) -> (164.257, 40.8838)
  line L674 (164.257, 40.8838) -> (164.257, 41.8828)
  line L675 (164.257, 41.8828) -> (165.056, 41.8828)
  line L676 (165.056, 41.8828) -> (165.056, 44.9834)
  line L677 (165.056, 44.9834) -> (164.257, 44.9834)
  line L678 (164.257, 44.9834) -> (164.257, 50.7834)
  line L679 (164.257, 50.7834) -> (165.056, 50.7834)
  line L680 (165.056, 50.7834) -> (165.056, 53.8826)
  line L681 (165.056, 53.8826) -> (164.257, 53.8826)
  line L682 (164.257, 53.8826) -> (164.257, 54.8831)
  line L683 (164.257, 54.8831) -> (150.257, 54.8831)
  line L684 (131.207, 54.8831) -> (131.207, 53.8826)
  line L685 (131.207, 53.8826) -> (130.406, 53.8826)
  line L686 (130.406, 53.8826) -> (130.406, 50.7834)
  line L687 (130.406, 50.7834) -> (131.207, 50.7834)
  line L688 (131.207, 50.7834) -> (131.207, 44.9834)
  line L689 (131.207, 44.9834) -> (130.406, 44.9834)
  line L690 (130.406, 44.9834) -> (130.406, 41.8828)
  line L691 (130.406, 41.8828) -> (131.207, 41.8828)
  line L692 (131.207, 41.8828) -> (131.207, 40.8838)
  line L693 (131.207, 40.8838) -> (145.207, 40.8838)
  line L694 (145.207, 40.8838) -> (145.207, 41.8828)
  line L695 (145.207, 41.8828) -> (146.006, 41.8828)
  line L696 (146.006, 41.8828) -> (146.006, 44.9834)
  line L697 (146.006, 44.9834) -> (145.207, 44.9834)
  line L698 (145.207, 44.9834) -> (145.207, 50.7834)
  line L699 (145.207, 50.7834) -> (146.006, 50.7834)
  line L700 (146.006, 50.7834) -> (146.006, 53.8826)
  line L701 (146.006, 53.8826) -> (145.207, 53.8826)
  line L702 (145.207, 53.8826) -> (145.207, 54.8831)
  line L703 (145.207, 54.8831) -> (131.207, 54.8831)
  line L704 (112.157, 54.8831) -> (112.157, 53.8826)
  line L705 (112.157, 53.8826) -> (111.356, 53.8826)
  line L706 (111.356, 53.8826) -> (111.356, 50.7834)
  line L707 (111.356, 50.7834) -> (112.157, 50.7834)
  line L708 (112.157, 50.7834) -> (112.157, 44.9834)
  line L709 (112.157, 44.9834) -> (111.356, 44.9834)
  line L710 (111.356, 44.9834) -> (111.356, 41.8828)
  line L711 (111.356, 41.8828) -> (112.157, 41.8828)
  line L712 (112.157, 41.8828) -> (112.157, 40.8838)
  line L713 (112.157, 40.8838) -> (126.157, 40.8838)
  line L714 (126.157, 40.8838) -> (126.157, 41.8828)
  line L715 (126.157, 41.8828) -> (126.956, 41.8828)
  line L716 (126.956, 41.8828) -> (126.956, 44.9834)
  line L717 (126.956, 44.9834) -> (126.157, 44.9834)
  line L718 (126.157, 44.9834) -> (126.157, 50.7834)
  line L719 (126.157, 50.7834) -> (126.956, 50.7834)
  line L720 (126.956, 50.7834) -> (126.956, 53.8826)
  line L721 (126.956, 53.8826) -> (126.157, 53.8826)
  line L722 (126.157, 53.8826) -> (126.157, 54.8831)
  line L723 (126.157, 54.8831) -> (112.157, 54.8831)
  line L724 (93.1072, 54.8831) -> (93.1072, 53.8826)
  line L725 (93.1072, 53.8826) -> (92.3064, 53.8826)
  line L726 (92.3064, 53.8826) -> (92.3064, 50.7834)
  line L727 (92.3064, 50.7834) -> (93.1072, 50.7834)
  line L728 (93.1072, 50.7834) -> (93.1072, 44.9834)
  line L729 (93.1072, 44.9834) -> (92.3064, 44.9834)
  line L730 (92.3064, 44.9834) -> (92.3064, 41.8828)
  line L731 (92.3064, 41.8828) -> (93.1072, 41.8828)
  line L732 (93.1072, 41.8828) -> (93.1072, 40.8838)
  line L733 (93.1072, 40.8838) -> (107.107, 40.8838)
  line L734 (107.107, 40.8838) -> (107.107, 41.8828)
  line L735 (107.107, 41.8828) -> (107.906, 41.8828)
  line L736 (107.906, 41.8828) -> (107.906, 44.9834)
  line L737 (107.906, 44.9834) -> (107.107, 44.9834)
  line L738 (107.107, 44.9834) -> (107.107, 50.7834)
  line L739 (107.107, 50.7834) -> (107.906, 50.7834)
  line L740 (107.906, 50.7834) -> (107.906, 53.8826)
  line L741 (107.906, 53.8826) -> (107.107, 53.8826)
  line L742 (107.107, 53.8826) -> (107.107, 54.8831)
  line L743 (107.107, 54.8831) -> (93.1072, 54.8831)
  line L744 (74.0572, 54.8831) -> (74.0572, 53.8826)
  line L745 (74.0572, 53.8826) -> (73.2564, 53.8826)
  line L746 (73.2564, 53.8826) -> (73.2564, 50.7834)
  line L747 (73.2564, 50.7834) -> (74.0572, 50.7834)
  line L748 (74.0572, 50.7834) -> (74.0572, 44.9834)
  line L749 (74.0572, 44.9834) -> (73.2564, 44.9834)
  line L750 (73.2564, 44.9834) -> (73.2564, 41.8828)
  line L751 (73.2564, 41.8828) -> (74.0572, 41.8828)
  line L752 (74.0572, 41.8828) -> (74.0572, 40.8838)
  line L753 (74.0572, 40.8838) -> (88.0565, 40.8838)
  line L754 (88.0565, 40.8838) -> (88.0565, 41.8828)
  line L755 (88.0565, 41.8828) -> (88.8559, 41.8828)
  line L756 (88.8559, 41.8828) -> (88.8559, 44.9834)
  line L757 (88.8559, 44.9834) -> (88.0565, 44.9834)
  line L758 (88.0565, 44.9834) -> (88.0565, 50.7834)
  line L759 (88.0565, 50.7834) -> (88.8559, 50.7834)
  line L760 (88.8559, 50.7834) -> (88.8559, 53.8826)
  line L761 (88.8559, 53.8826) -> (88.0565, 53.8826)
  line L762 (88.0565, 53.8826) -> (88.0565, 54.8831)
  line L763 (88.0565, 54.8831) -> (74.0572, 54.8831)
  line L764 (55.0072, 54.8831) -> (55.0072, 53.8826)
  line L765 (55.0072, 53.8826) -> (54.2064, 53.8826)
  line L766 (54.2064, 53.8826) -> (54.2064, 50.7834)
  line L767 (54.2064, 50.7834) -> (55.0072, 50.7834)
  line L768 (55.0072, 50.7834) -> (55.0072, 44.9834)
  line L769 (55.0072, 44.9834) -> (54.2064, 44.9834)
  line L770 (54.2064, 44.9834) -> (54.2064, 41.8828)
  line L771 (54.2064, 41.8828) -> (55.0072, 41.8828)
  line L772 (55.0072, 41.8828) -> (55.0072, 40.8838)
  line L773 (55.0072, 40.8838) -> (69.0065, 40.8838)
  line L774 (69.0065, 40.8838) -> (69.0065, 41.8828)
  line L775 (69.0065, 41.8828) -> (69.8059, 41.8828)
  line L776 (69.8059, 41.8828) -> (69.8059, 44.9834)
  line L777 (69.8059, 44.9834) -> (69.0065, 44.9834)
  line L778 (69.0065, 44.9834) -> (69.0065, 50.7834)
  line L779 (69.0065, 50.7834) -> (69.8059, 50.7834)
  line L780 (69.8059, 50.7834) -> (69.8059, 53.8826)
  line L781 (69.8059, 53.8826) -> (69.0065, 53.8826)
  line L782 (69.0065, 53.8826) -> (69.0065, 54.8831)
  line L783 (69.0065, 54.8831) -> (55.0072, 54.8831)
  line L784 (35.9572, 54.8831) -> (35.9572, 53.8826)
  line L785 (35.9572, 53.8826) -> (35.1565, 53.8826)
  line L786 (35.1565, 53.8826) -> (35.1565, 50.7834)
  line L787 (35.1565, 50.7834) -> (35.9572, 50.7834)
  line L788 (35.9572, 50.7834) -> (35.9572, 44.9834)
  line L789 (35.9572, 44.9834) -> (35.1565, 44.9834)
  line L790 (35.1565, 44.9834) -> (35.1565, 41.8828)
  line L791 (35.1565, 41.8828) -> (35.9572, 41.8828)
  line L792 (35.9572, 41.8828) -> (35.9572, 40.8838)
  line L793 (35.9572, 40.8838) -> (49.9565, 40.8838)
  line L794 (49.9565, 40.8838) -> (49.9565, 41.8828)
  line L795 (49.9565, 41.8828) -> (50.7559, 41.8828)
  line L796 (50.7559, 41.8828) -> (50.7559, 44.9834)
  line L797 (50.7559, 44.9834) -> (49.9565, 44.9834)
  line L798 (49.9565, 44.9834) -> (49.9565, 50.7834)
  line L799 (49.9565, 50.7834) -> (50.7559, 50.7834)
  line L800 (50.7559, 50.7834) -> (50.7559, 53.8826)
  line L801 (50.7559, 53.8826) -> (49.9565, 53.8826)
  line L802 (49.9565, 53.8826) -> (49.9565, 54.8831)
  line L803 (49.9565, 54.8831) -> (35.9572, 54.8831)
  line L804 (9.762, 54.8831) -> (9.762, 53.8826)
  line L805 (9.762, 53.8826) -> (8.9628, 53.8826)
  line L806 (8.9628, 53.8826) -> (8.9628, 50.7834)
  line L807 (8.9628, 50.7834) -> (9.762, 50.7834)
  line L808 (9.762, 50.7834) -> (9.762, 44.9834)
  line L809 (9.762, 44.9834) -> (8.9628, 44.9834)
  line L810 (8.9628, 44.9834) -> (8.9628, 41.8828)
  line L811 (8.9628, 41.8828) -> (9.762, 41.8828)
  line L812 (9.762, 41.8828) -> (9.762, 40.8838)
  line L813 (9.762, 40.8838) -> (23.7629, 40.8838)
  line L814 (23.7629, 40.8838) -> (23.7629, 41.8828)
  line L815 (23.7629, 41.8828) -> (24.5622, 41.8828)
  line L816 (24.5622, 41.8828) -> (24.5622, 44.9834)
  line L817 (24.5622, 44.9834) -> (23.7629, 44.9834)
  line L818 (23.7629, 44.9834) -> (23.7629, 50.7834)
  line L819 (23.7629, 50.7834) -> (24.5622, 50.7834)
  line L820 (24.5622, 50.7834) -> (24.5622, 53.8826)
  line L821 (24.5622, 53.8826) -> (23.7629, 53.8826)
  line L822 (23.7629, 53.8826) -> (23.7629, 54.8831)
  line L823 (23.7629, 54.8831) -> (9.762, 54.8831)
  line L824 (264.557, 73.9331) -> (264.557, 72.9326)
  line L825 (264.557, 72.9326) -> (263.756, 72.9326)
  line L826 (263.756, 72.9326) -> (263.756, 69.8334)
  line L827 (263.756, 69.8334) -> (264.557, 69.8334)
  line L828 (264.557, 69.8334) -> (264.557, 64.0334)
  line L829 (264.557, 64.0334) -> (263.756, 64.0334)
  line L830 (263.756, 64.0334) -> (263.756, 60.9328)
  line L831 (263.756, 60.9328) -> (264.557, 60.9328)
  line L832 (264.557, 60.9328) -> (264.557, 59.9338)
  line L833 (264.557, 59.9338) -> (278.557, 59.9338)
  line L834 (278.557, 59.9338) -> (278.557, 60.9328)
  line L835 (278.557, 60.9328) -> (279.356, 60.9328)
  line L836 (279.356, 60.9328) -> (279.356, 64.0334)
  line L837 (279.356, 64.0334) -> (278.557, 64.0334)
  line L838 (278.557, 64.0334) -> (278.557, 69.8334)
  line L839 (278.557, 69.8334) -> (279.356, 69.8334)
  line L840 (279.356, 69.8334) -> (279.356, 72.9326)
  line L841 (279.356, 72.9326) -> (278.557, 72.9326)
  line L842 (278.557, 72.9326) -> (278.557, 73.9331)
  line L843 (278.557, 73.9331) -> (264.557, 73.9331)
  line L844 (240.745, 73.9331) -> (240.745, 72.9326)
  line L845 (240.745, 72.9326) -> (239.944, 72.9326)
  line L846 (239.944, 72.9326) -> (239.944, 69.8334)
  line L847 (239.944, 69.8334) -> (240.745, 69.8334)
  line L848 (240.745, 69.8334) -> (240.745, 64.0334)
  line L849 (240.745, 64.0334) -> (239.944, 64.0334)
  line L850 (239.944, 64.0334) -> (239.944, 60.9328)
  line L851 (239.944, 60.9328) -> (240.745, 60.9328)
  line L852 (240.745, 60.9328) -> (240.745, 59.9338)
  line L853 (240.745, 59.9338) -> (254.744, 59.9338)
  line L854 (254.744, 59.9338) -> (254.744, 60.9328)
  line L855 (254.744, 60.9328) -> (255.545, 60.9328)
  line L856 (255.545, 60.9328) -> (255.545, 64.0334)
  line L857 (255.545, 64.0334) -> (254.744, 64.0334)
  line L858 (254.744, 64.0334) -> (254.744, 69.8334)
  line L859 (254.744, 69.8334) -> (255.545, 69.8334)
  line L860 (255.545, 69.8334) -> (255.545, 72.9326)
  line L861 (255.545, 72.9326) -> (254.744, 72.9326)
  line L862 (254.744, 72.9326) -> (254.744, 73.9331)
  line L863 (254.744, 73.9331) -> (240.745, 73.9331)
  line L864 (221.695, 73.9331) -> (221.695, 72.9326)
  line L865 (221.695, 72.9326) -> (220.894, 72.9326)
  line L866 (220.894, 72.9326) -> (220.894, 69.8334)
  line L867 (220.894, 69.8334) -> (221.695, 69.8334)
  line L868 (221.695, 69.8334) -> (221.695, 64.0334)
  line L869 (221.695, 64.0334) -> (220.894, 64.0334)
  line L870 (220.894, 64.0334) -> (220.894, 60.9328)
  line L871 (220.894, 60.9328) -> (221.695, 60.9328)
  line L872 (221.695, 60.9328) -> (221.695, 59.9338)
  line L873 (221.695, 59.9338) -> (235.694, 59.9338)
  line L874 (235.694, 59.9338) -> (235.694, 60.9328)
  line L875 (235.694, 60.9328) -> (236.495, 60.9328)
  line L876 (236.495, 60.9328) -> (236.495, 64.0334)
  line L877 (236.495, 64.0334) -> (235.694, 64.0334)
  line L878 (235.694, 64.0334) -> (235.694, 69.8334)
  line L879 (235.694, 69.8334) -> (236.495, 69.8334)
  line L880 (236.495, 69.8334) -> (236.495, 72.9326)
  line L881 (236.495, 72.9326) -> (235.694, 72.9326)
  line L882 (235.694, 72.9326) -> (235.694, 73.9331)
  line L883 (235.694, 73.9331) -> (221.695, 73.9331)
  line L884 (202.645, 73.9331) -> (202.645, 72.9326)
  line L885 (202.645, 72.9326) -> (201.844, 72.9326)
  line L886 (201.844, 72.9326) -> (201.844, 69.8334)
  line L887 (201.844, 69.8334) -> (202.645, 69.8334)
  line L888 (202.645, 69.8334) -> (202.645, 64.0334)
  line L889 (202.645, 64.0334) -> (201.844, 64.0334)
  line L890 (201.844, 64.0334) -> (201.844, 60.9328)
  line L891 (201.844, 60.9328) -> (202.645, 60.9328)
  line L892 (202.645, 60.9328) -> (202.645, 59.9338)
  line L893 (202.645, 59.9338) -> (216.644, 59.9338)
  line L894 (216.644, 59.9338) -> (216.644, 60.9328)
  line L895 (216.644, 60.9328) -> (217.445, 60.9328)
  line L896 (217.445, 60.9328) -> (217.445, 64.0334)
  line L897 (217.445, 64.0334) -> (216.644, 64.0334)
  line L898 (216.644, 64.0334) -> (216.644, 69.8334)
  line L899 (216.644, 69.8334) -> (217.445, 69.8334)
  line L900 (217.445, 69.8334) -> (217.445, 72.9326)
  line L901 (217.445, 72.9326) -> (216.644, 72.9326)
  line L902 (216.644, 72.9326) -> (216.644, 73.9331)
  line L903 (216.644, 73.9331) -> (202.645, 73.9331)
  line L904 (183.595, 73.9331) -> (183.595, 72.9326)
  line L905 (183.595, 72.9326) -> (182.794, 72.9326)
  line L906 (182.794, 72.9326) -> (182.794, 69.8334)
  line L907 (182.794, 69.8334) -> (183.595, 69.8334)
  line L908 (183.595, 69.8334) -> (183.595, 64.0334)
  line L909 (183.595, 64.0334) -> (182.794, 64.0334)
  line L910 (182.794, 64.0334) -> (182.794, 60.9328)
  line L911 (182.794, 60.9328) -> (183.595, 60.9328)
  line L912 (183.595, 60.9328) -> (183.595, 59.9338)
  line L913 (183.595, 59.9338) -> (197.594, 59.9338)
  line L914 (197.594, 59.9338) -> (197.594, 60.9328)
  line L915 (197.594, 60.9328) -> (198.395, 60.9328)
  line L916 (198.395, 60.9328) -> (198.395, 64.0334)
  line L917 (198.395, 64.0334) -> (197.594, 64.0334)
  line L918 (197.594, 64.0334) -> (197.594, 69.8334)
  line L919 (197.594, 69.8334) -> (198.395, 69.8334)
  line L920 (198.395, 69.8334) -> (198.395, 72.9326)
  line L921 (198.395, 72.9326) -> (197.594, 72.9326)
  line L922 (197.594, 72.9326) -> (197.594, 73.9331)
  line L923 (197.594, 73.9331) -> (183.595, 73.9331)
  line L924 (164.545, 73.9331) -> (164.545, 72.9326)
  line L925 (164.545, 72.9326) -> (163.744, 72.9326)
  line L926 (163.744, 72.9326) -> (163.744, 69.8334)
  line L927 (163.744, 69.8334) -> (164.545, 69.8334)
  line L928 (164.545, 69.8334) -> (164.545, 64.0334)
  line L929 (164.545, 64.0334) -> (163.744, 64.0334)
  line L930 (163.744, 64.0334) -> (163.744, 60.9328)
  line L931 (163.744, 60.9328) -> (164.545, 60.9328)
  line L932 (164.545, 60.9328) -> (164.545, 59.9338)
  line L933 (164.545, 59.9338) -> (178.544, 59.9338)
  line L934 (178.544, 59.9338) -> (178.544, 60.9328)
  line L935 (178.544, 60.9328) -> (179.345, 60.9328)
  line L936 (179.345, 60.9328) -> (179.345, 64.0334)
  line L937 (179.345, 64.0334) -> (178.544, 64.0334)
  line L938 (178.544, 64.0334) -> (178.544, 69.8334)
  line L939 (178.544, 69.8334) -> (179.345, 69.8334)
  line L940 (179.345, 69.8334) -> (179.345, 72.9326)
  line L941 (179.345, 72.9326) -> (178.544, 72.9326)
  line L942 (178.544, 72.9326) -> (178.544, 73.9331)